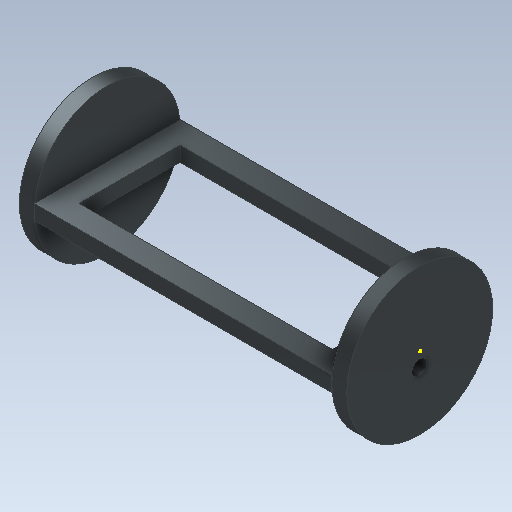
# Autodesk Inventor part: electronicsbay
Saved by Autodesk Inventor 2020.3 (Build 243373000, 373)
## iProperties
Created: 2021-03-10
Part Number: electronicsbay
Material: ABS Plastic
Document SubType Name: Modeling
Designer: 0x6f736f646f
Density: 1.06 g/cm^3
Appearance: Iron Gray
Author: 0x6f736f646f
Autodesk Inventor part; units mm, degrees
ref_plane "YZ Plane" through (0, 0, 0) normal (1, 0, 0) x (0, 1, 0)
ref_plane "XZ Plane" through (0, 0, 0) normal (0, 1, 0) x (-1, 0, 0)
ref_plane "XY Plane" through (0, 0, 0) normal (0, 0, 1) x (1, 0, 0)
sketch "Sketch1" plane through (0, 0, 0) normal (0, 1, 0) x (-1, 0, 0)
  point P0 (0, 0)
sketch "Sketch2" plane through (0, 0, 0) normal (0, 0, 1) x (1, 0, 0)
  line L0 (0, 0) -> (0, 24.5)
  line L1 (0, 24.5) -> (-5, 24.5)
  line L2 (-5, 24.5) -> (-5, 2.5)
  line L3 (-5, 2.5) -> (-105, 2.5)
  line L4 (-105, 2.5) -> (-105, 24.5)
  line L5 (-105, 24.5) -> (-110, 24.5)
  line L6 (-110, 24.5) -> (-110, 0)
  line L7 (-110, 0) -> (0, 0)
  line L8 (-105, 2.5) -> (-5, 2.5)
  line L9 (-5, 2.5) -> (-5, -2.5)
  line L10 (-5, -2.5) -> (-105, -2.5)
  line L11 (-105, -2.5) -> (-105, 2.5)
  point P0 (-5, 2.5)
  dimension "d0" = 24.5
  dimension "d1" = 5
  dimension "d2" = 22
  dimension "d3" = 100
  dimension "d4" = 5
  dimension "d6" = 5
  constraints: 24 end point, 7 perpendicular, 2 parallel, 2 point on line, 1 horizontal, 1 vertical
  measures "d0" distance of L0.start L0.end
  measures "d1" distance of L0.end L1.end
  measures "d2" distance of L1.end L2.end
  measures "d3" distance of L2.end L3.end
  measures "d4" distance of L4.end L5.end
  measures "d6" distance of L8.end L9.end
revolve "Revolution1" add sketch "Sketch2" angle 360 about axis through (-110, 0, 0) along (1, 0, 0) contours L7 L9 L2 L1 L0 | L7 L11 L3 L9 | L7 L6 L5 L4 L11
extrude "Extrusion1" add sketch "Sketch2" along normal mid plane 49 contours L9 L10 L11 L7 | L7 L11 L3 L9
sketch "Sketch3" plane through (-105, 2.5, -24.5) normal (0, 1, 0) x (1, 0, 0)
  line L0 (100, 0) -> (0, 0) projected
  line L1 (100, -48.8721) -> (100, -0.1279) projected
  line L2 (0, 0) -> (100, 0)
  line L3 (100, 0) -> (100, -48.8721)
  line L4 (100, -48.8721) -> (0, -48.8721)
  line L5 (0, -48.8721) -> (0, 0)
  line L6 (7.5, -7.5) -> (92.5, -7.5)
  line L7 (92.5, -7.5) -> (92.5, -41.3721)
  line L8 (92.5, -41.3721) -> (7.5, -41.3721)
  line L9 (7.5, -41.3721) -> (7.5, -7.5)
  point P0 (105, -24.5)
  dimension "d9" = 7.5
  constraints: 16 end point, 4 parallel, 2 perpendicular, 1 horizontal, 3 other
  measures "d9" distance between parallel lines of L5 L9
extrude "Extrusion2" cut sketch "Sketch3" against normal mid plane 20 contours L6 L7 L8 L9
sketch "Sketch4" plane through (0, 0, 0) normal (1, 0, 0) x (0, 1, 0)
  circle A0 centre (-5, 0) radius 2.5
  point P0 (0, 0)
  dimension "d13" = 5
  dimension "d16" = 5
  constraints: 1 centre point
  measures "d13" diameter of A0
  measures "d16" distance of A0.centre point (0, 0)
extrude "Extrusion3" cut sketch "Sketch4" against normal blind 10
body "Solid1"
